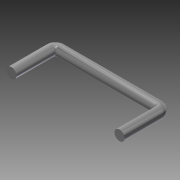
# Autodesk Inventor part: handle
Saved by Autodesk Inventor 2014 SP2 (Build 180246200, 246)
## iProperties
Created: 2016-09-20
Part Number: handle
Material: Stainless Steel, Austenitic
Document SubType Name: Modeling
Designer: cruiser
Density: 8.03 g/cm^3
Appearance: Semi-Polished
Mass: 12.8786 g
Surface Area: 13.8266 cm^2
Volume: 1.6038 cm^3
Author: cruiser
Autodesk Inventor part; units mm, degrees
ref_plane "YZ Plane" through (0, 0, 0) normal (1, 0, 0) x (0, 1, 0)
ref_plane "XZ Plane" through (0, 0, 0) normal (0, 1, 0) x (-1, 0, 0)
ref_plane "XY Plane" through (0, 0, 0) normal (0, 0, 1) x (1, 0, 0)
sketch "Sketch1" plane through (0, 0, 0) normal (0, 0, 1) x (1, 0, 0)
  line L0 (-50.8, 0) -> (-50.8, 18.2562)
  line L1 (-48.4188, 20.6375) -> (-2.3813, 20.6375)
  line L2 (0, 18.2562) -> (0, 0)
  arc A0 (-48.4188, 20.6375) -> (-50.8, 18.2562) centre (-48.4188, 18.2562) ccw
  arc A1 (0, 18.2562) -> (-2.3813, 20.6375) centre (-2.3813, 18.2562) ccw
  line L3 (0, 0) -> (0, 63.2917)
  point P0 (-50.8, 20.6375)
  point P1 (0, 20.6375)
  dimension "d0" = 20.6375
  dimension "d1" = 50.8
  dimension "d2" = 2.3813
  dimension "d4" = 90
  dimension "d6" = 0
  dimension "d7" = 20.6375
  constraints: 8 end point, 4 point on circle, 4 point on line, 4 tangent, 2 centre point, 1 equal radius, 1 parallel, 1 vertical
  measures "d0" distance of L0.start point (-50.8, 20.637)
  measures "d1" distance of point (-50.8, 20.637) point (0, 20.638)
  measures "d2" radius of A0
  measures "d4" angle of L2 L1
  measures "d6" distance between parallel lines of L2 L3
  measures "d7" distance from line of L2.end L1
sketch "Sketch2" plane through (0, 0, 0) normal (0, 1, 0) x (-1, 0, 0)
  circle A0 centre (0, 0) radius 2.3813
  dimension "d3" = 4.7625
  constraints: 1 centre point, 1 coincident
  measures "d3" diameter of A0
sweep "Sweep1" add profiles "Sketch2" path "Sketch1" path curves L2 A1 L1 A0 L0
equation "\"d0\" = handle_projection"
equation "\"d1\" = handle_spacing"
equation "\"d2\" = 0.5 * handle_d"
equation "\"d7\" = handle_projection"
equation "\"d3\" = handle_d"
equation "\"laserresin\" = 5"
equation "\"st1_thickness\" = 0.91186"
equation "\"st2_thickness\" = 1.5875"
equation "\"st3_thickness\" = 1.5875"
equation "\"al1_thickness\" = 0.79375"
equation "\"al2_thickness\" = 1.5875"
equation "\"al3_thickness\" = 1.5875"
equation "\"bend_factor\" = 2.26205"
equation "\"st1_bend\" = 2.06267"
equation "\"st2_bend\" = 3.591"
equation "\"st3_bend\" = 3.591"
equation "\"al1_bend\" = 1.7955"
equation "\"al2_bend\" = 3.591"
equation "\"al3_bend\" = 3.591"
equation "\"acrylic1_thickness\" = 5.88"
equation "\"acrylic2_thickness\" = 3.15"
equation "\"acrylic3_thickness\" = 3.15"
equation "\"linear_bearing_spacing\" = 208.23622"
equation "\"nema17_x\" = 43"
equation "\"nema17_shaft\" = 24"
equation "\"lmk8uu_x\" = 25"
equation "\"lmk8uu_shaft\" = 15"
equation "\"lmk8uu_z\" = 24"
equation "\"shf8_y\" = 43"
equation "\"acme_nut_d\" = 19.1"
equation "\"acme_nut_upper_d\" = 12.7"
equation "\"handle_spacing\" = 50.8"
equation "\"handle_hole_d\" = 5.0625"
equation "\"handle_projection\" = 20.6375"
equation "\"switch_spacing\" = 19"
equation "\"laser_body_diameter\" = 12"
equation "\"m3_diameter\" = 3"
equation "\"m3_head\" = 6"
equation "\"m4_diameter\" = 4"
equation "\"m5_diameter\" = 5"
equation "\"m5_head\" = 10.3"
equation "\"rivet_diameter\" = 3.3"
equation "\"brass_insert_drill\" = 4"
equation "\"m5_brass_insert_drill\" = 6.7"
equation "\"m3_press_nut_drill\" = 4.5"
equation "\"m5_press_nut_drill\" = 6.5"
equation "\"platform_t\" = 1.5875"
equation "\"platform_fold_x\" = 25"
equation "\"platform_crane_gap\" = 0.1"
equation "\"platform_upper_y\" = 46.625"
equation "\"crane_t\" = 1.5875"
equation "\"crane_x\" = 233.23622"
equation "\"crane_gap\" = 0.1"
equation "\"tray_t\" = 5.88"
equation "\"tray_to_platform_oversize\" = 0"
equation "\"reservoir_t\" = 0.79375"
equation "\"reservoir_flap_y\" = 20.79375"
equation "\"frame_front_t\" = 0.91186"
equation "\"frame_front_x\" = 280.23622"
equation "\"frame_front_y\" = 56"
equation "\"frame_front_fold\" = 15"
equation "\"frame_gap\" = 0.1"
equation "\"frame_back_t\" = 0.91186"
equation "\"frame_back_x\" = 278.2125"
equation "\"frame_back_y\" = 53.97628"
equation "\"frame_back_z\" = 497.97628"
equation "\"frame_opening_x\" = 200.23622"
equation "\"drawer_t\" = 0.79375"
equation "\"drawer_gap\" = 0.1"
equation "\"drawer_reservoir_overlap_x\" = 24.20625"
equation "\"drawer_x\" = 202.02372"
equation "\"drawer_y\" = 72"
equation "\"drawer_window_gap\" = 5"
equation "\"foot_t\" = 0.91186"
equation "\"foot_x\" = 202.02372"
equation "\"foot_z\" = 15"
equation "\"handle_d\" = 4.7625"
equation "\"laser_holder_t\" = 0.79375"
equation "\"laser_holder_z\" = 75"
equation "\"laser_offset_x\" = 59.11811"
equation "\"subframe_x\" = 66"
equation "\"subframe_t\" = 0.79375"
equation "\"subframe_y\" = 55"
equation "\"laser_offset_y\" = 8.5"
equation "\"galvo_y_in_offset\" = 17.5"
equation "\"galvo_y_out_offset\" = 27"
equation "\"laser_diameter\" = 13"
equation "\"corner_small_r\" = 1"
equation "\"corner_big_r\" = 5"
equation "\"rivet1_diameter\" = 3.26"
equation "\"rivet2_diameter\" = 3.26"
body "Solid1"
